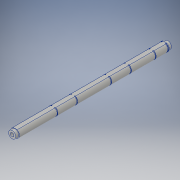
# Autodesk Inventor part: Column Axle
Saved by Autodesk Inventor 2019.4 (Build 234330000, 330)
## iProperties
Created: 2020-01-23
Part Number: Column Axle
Material: Aluminum 6061
Document SubType Name: Modeling
Designer: admin
Density: 2.7 g/cm^3
Appearance: Aluminum - Flat
Mass: 53.1021 g
Surface Area: 120.089 cm^2
Volume: 19.6675 cm^3
Author: admin
Autodesk Inventor part; units mm, degrees
ref_plane "YZ Plane" through (0, 0, 0) normal (1, 0, 0) x (0, 1, 0)
ref_plane "XZ Plane" through (0, 0, 0) normal (0, 1, 0) x (-1, 0, 0)
ref_plane "XY Plane" through (0, 0, 0) normal (0, 0, 1) x (1, 0, 0)
sketch "Sketch1" plane through (0, 0, 0) normal (1, 0, 0) x (0, 1, 0)
  line L0 (0, 0) -> (5, 0)
  line L1 (5, 0) -> (5, -4)
  line L2 (5, -4) -> (6, -4)
  line L3 (6, -4) -> (6, -4.9)
  line L4 (6, -4.9) -> (6, -4.9)
  line L5 (6, -4.9) -> (6, -6)
  line L6 (6, -6) -> (6, -6)
  line L7 (6, -6) -> (6, -18.649)
  line L8 (6, -18.649) -> (6, -18.649)
  line L9 (6, -55.9) -> (5.65, -55.9)
  line L10 (5.65, -55.9) -> (5.65, -57)
  line L11 (5.65, -57) -> (6, -57)
  line L12 (6, -57) -> (6, -83)
  line L13 (6, -83) -> (5.65, -83)
  line L14 (5.65, -83) -> (5.65, -84.1)
  line L15 (5.65, -84.1) -> (6, -84.1)
  line L16 (6, -84.1) -> (6, -129.9)
  line L17 (6, -129.9) -> (5.65, -129.9)
  line L18 (5.65, -129.9) -> (5.65, -131)
  line L19 (5.65, -131) -> (6, -131)
  line L20 (6, -131) -> (6, -157)
  line L21 (6, -157) -> (5.65, -157)
  line L22 (5.65, -157) -> (5.65, -158.1)
  line L23 (5.65, -158.1) -> (6, -158.1)
  line L24 (6, -158.1) -> (6, -190.9)
  line L25 (6, -190.9) -> (5.65, -190.9)
  line L26 (5.65, -190.9) -> (5.65, -192)
  line L27 (5.65, -192) -> (6, -192)
  line L28 (6, -192) -> (6, -208)
  line L29 (6, -208) -> (5.65, -208)
  line L30 (5.65, -208) -> (5.65, -209.1)
  line L31 (5.65, -209.1) -> (6, -209.1)
  line L32 (6, -209.1) -> (6, -210)
  line L33 (6, -210) -> (5, -210)
  line L34 (5, -210) -> (5, -214)
  line L35 (5, -214) -> (0, -214)
  line L36 (0, -214) -> (0, 0)
  line L37 (6, -18.649) -> (6, -19.749)
  line L38 (6, -19.749) -> (6, -19.749)
  line L39 (6, -19.749) -> (6, -55.9)
  dimension "d0" = 5
  dimension "d1" = 6
  dimension "d2" = 0
  dimension "d4" = 0.35
  dimension "d5" = 1.1
  dimension "d6" = 1.1
  dimension "d7" = 1.1
  dimension "d8" = 1.1
  dimension "d9" = 1.1
  dimension "d10" = 1.1
  dimension "d11" = 4
  dimension "d12" = 1.1
  dimension "d13" = 2
  dimension "d14" = 5
  dimension "d15" = 12.649
  dimension "d16" = 4
  dimension "d17" = 0
  dimension "d18" = 1.1
  dimension "d19" = 6
  dimension "d20" = 26
  dimension "d21" = 16
  dimension "d23" = 26
  dimension "d24" = 57
  dimension "d26" = 2
  dimension "d35" = 57
  dimension "d36" = 206
  constraints: 80 end point, 25 perpendicular, 22 point on line, 2 vertical, 1 collinear, 1 horizontal
  measures "d0" distance of L0.start L0.end
  measures "d1" distance between parallel lines of L36 L7
  measures "d2" distance of L5.end L6.end
  measures "d4" distance of L9.start L9.end
  measures "d5" distance of L9.end L10.end
  measures "d6" distance of L13.end L14.end
  measures "d7" distance of L17.end L18.end
  measures "d8" distance of L21.end L22.end
  measures "d9" distance of L25.end L26.end
  measures "d10" distance of L29.end L30.end
  measures "d11" distance of L0.end L1.end
  measures "d12" distance of L4.end L5.end
  measures "d13" distance between parallel lines of L2 L6
  measures "d14" distance between parallel lines of L36 L34
  measures "d15" distance of L6.end L7.end
  measures "d16" distance of L33.end L34.end
  measures "d17" distance of L37.end L38.end
  measures "d18" distance of L8.end L37.end
  measures "d19" distance between parallel lines of L36 L12
  measures "d20" distance of L11.end L12.end
  measures "d21" distance of L27.end L28.end
  measures "d23" distance of L19.end L20.end
  measures "d24" distance between parallel lines of L0 L11
  measures "d26" distance between parallel lines of L33 L29
  measures "d35" distance between parallel lines of L35 L21
  measures "d36" distance between parallel lines of L33 L2
revolve "Revolution1" add sketch "Sketch1" angle 360 about axis through (0, 0, -214) along (0, 0, 1)
sketch "Sketch2" plane through (0, 0, 0) normal (0, 0, 1) x (1, 0, 0)
  circle A0 centre (0, 0) radius 5 projected
  point P0 (0, 0)
  constraints: 1 coincident
hole "Hole1" at (0, 0, 0) direction (0, 0, -1) diameter 5 end through all
sketch "Sketch3" plane through (0, 0, -18.649) normal (0, 0, -1) x (-1, 0, 0)
  line L0 (0, 7.1591) -> (6.2, 3.5796)
  line L1 (6.2, 3.5796) -> (6.2, -3.5796)
  line L2 (6.2, -3.5796) -> (0, -7.1591)
  line L3 (0, -7.1591) -> (-6.2, -3.5796)
  line L4 (-6.2, -3.5796) -> (-6.2, 3.5796)
  line L5 (-6.2, 3.5796) -> (0, 7.1591)
  circle A0 centre (0, 0) radius 7.5 projected
  point P0 (0, 0)
  point P1 (0, 0)
  dimension "d37" = 12.4
  constraints: 12 end point, 1 coincident, 13 other
  measures "d37" distance between parallel lines of L1 L4
extrude "Extrusion1" [suppressed]
sketch "Sketch4" plane through (0, 0, -55.9) normal (0, 0, 1) x (1, 0, 0)
  circle A0 centre (0, 0) radius 5.65 construction
  circle A1 centre (0, 0) radius 6 projected
  line L0 (-2.9047, 5.25) -> (2.9047, 5.25)
  point P0 (0, 0)
  dimension "d42" = 5.25
  constraints: 2 end point, 2 point on circle, 1 horizontal
  measures "d42" distance from line of A0.centre L0
extrude "Extrusion2" cut sketch "Sketch4" along normal through all both and the other way through all contours L0 A1 picked at (-0.2018, 5.4898)
body "Solid1"
